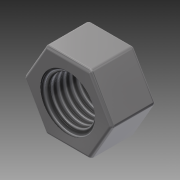
# Autodesk Inventor part: Pieza3
Saved by Autodesk Inventor 2013 (Build 170138000, 138)
## iProperties
Created: 2013-06-07
Part Number: Pieza3
Material: Acero
Document SubType Name: Modeling
Designer: BRAYAN
Density: 1 g/cm^3
Author: BRAYAN
Autodesk Inventor part; units mm, degrees
ref_plane "YZ Plane" through (0, 0, 0) normal (1, 0, 0) x (0, 1, 0)
ref_plane "XZ Plane" through (0, 0, 0) normal (0, 1, 0) x (-1, 0, 0)
ref_plane "XY Plane" through (0, 0, 0) normal (0, 0, 1) x (1, 0, 0)
sketch "Boceto1" plane through (0, 0, 0) normal (0, 1, 0) x (-1, 0, 0)
  line L0 (-5.5852, -5.9648) -> (1.4148, -5.9648)
  line L1 (1.4148, -5.9648) -> (4.9148, 0.0974)
  line L2 (4.9148, 0.0974) -> (1.4148, 6.1595)
  line L3 (1.4148, 6.1595) -> (-5.5852, 6.1595)
  line L4 (-5.5852, 6.1595) -> (-9.0852, 0.0974)
  line L5 (-9.0852, 0.0974) -> (-5.5852, -5.9648)
  circle A0 centre (-2.0852, 0.0974) radius 3.5
  dimension "d21" = 7
  dimension "d22" = 7
  dimension "d23" = 120
  dimension "d24" = 7
  dimension "d25" = 7
  dimension "d26" = 7
  dimension "d27" = 120
  dimension "d28" = 7
  constraints: 12 end point, 3 parallel, 1 centre point, 1 horizontal
  measures "d21" distance of L0.start L0.end
  measures "d22" distance of L0.end L1.end
  measures "d23" angle of L1 L0
  measures "d24" distance of L1.end L2.end
  measures "d25" distance of L2.end L3.end
  measures "d26" distance of L3.end L4.end
  measures "d27" angle of L4 L3
  measures "d28" diameter of A0
extrude "Extrusión1" add sketch "Boceto1" along normal blind 7
thread "Rosca1" size "M7x1" class "6H" standard "ANSI Metric M Profile" full length
fillet "Empalme1" radius 0.5 18 edges at (-1.4148, 3.5, 6.1595) (-4.9148, 3.5, 0.0974) (-1.4148, 3.5, -5.9648) (5.5852, 3.5, -5.9648) (9.0852, 3.5, 0.0974) (5.5852, 3.5, 6.1595) (7.3352, 0, 3.1284) (2.0852, 0, 6.1595) (-3.1648, 0, 3.1284) (-3.1648, 0, -2.9337) (2.0852, 0, -5.9648) (7.3352, 0, -2.9337) (7.3352, 7, 3.1284) (7.3352, 7, -2.9337) (2.0852, 7, -5.9648) (-3.1648, 7, -2.9337) (-3.1648, 7, 3.1284) (2.0852, 7, 6.1595)
chamfer "Chaflán1" distance 0.8 angle 45 2 edges at (5.5852, 7, 0.0974) (5.5852, 0, 0.0974)
thread "Rosca2" size "Rc 1/16" standard "ISO Taper Internal" full length
thread "Rosca3" size "Rc 1/16" standard "ISO Taper Internal" full length
